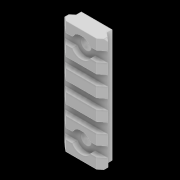
# Autodesk Inventor part: Picatinny6
Saved by Autodesk Inventor 2020.4 (Build 244396010, 396A)
## iProperties
Created: 2022-09-17
Part Number: Picatinny6
Material: Generic
Document SubType Name: Modeling
Designer: Val
Density: 1 g/cm^3
Appearance: Default
Author: Val
Autodesk Inventor part; units mm, degrees
ref_plane "YZ Plane" through (0, 0, 0) normal (1, 0, 0) x (0, 1, 0)
ref_plane "XZ Plane" through (0, 0, 0) normal (0, 1, 0) x (-1, 0, 0)
ref_plane "XY Plane" through (0, 0, 0) normal (0, 0, 1) x (1, 0, 0)
sketch "Base" plane through (0, 0, 0) normal (0, 0, 1) x (1, 0, 0)
  line L0 (-7.5, 55) -> (7.5, 55)
  line L1 (7.5, 55) -> (7.5, 0)
  line L2 (7.5, 0) -> (-7.5, 0)
  line L3 (-7.5, 0) -> (-7.5, 55)
  point P0 (0, 0)
  point P1 (0, 0)
  dimension "d0" = 55
  dimension "d1" = 15
  constraints: 8 end point, 2 parallel, 1 coincident, 1 horizontal, 1 midpoint, 1 perpendicular
  measures "d0" distance of L2.end L0.start
  measures "d1" distance of L0.start L0.end
extrude "BaseFeature" add sketch "Base" along normal blind 2.54
sketch "Profile" plane through (-7.5, 0, 0) normal (0, -1, 0) x (1, 0, 0)
  line L0 (0, 2.54) -> (15, 2.54) projected
  line L1 (0, 2.54) -> (15, 2.54)
  line L2 (15, 2.54) -> (15, 7.5692) construction
  line L3 (15, 7.5692) -> (0, 7.5692)
  line L4 (0, 7.5692) -> (0, 2.54) construction
  line L5 (-3.041, 5.0546) -> (18.041, 5.0546) construction
  line L6 (15, 7.5692) -> (18.041, 5.0546)
  line L7 (15, 2.54) -> (18.041, 5.0546)
  line L8 (0, 7.5692) -> (-3.041, 5.0546)
  line L9 (-3.041, 5.0546) -> (0, 2.54)
  point P0 (7.5, 0)
  point P1 (15, 5.0546)
  dimension "d4" = 5.0292
  dimension "d5" = 21.082
  constraints: 18 end point, 4 parallel, 2 horizontal, 1 midpoint, 1 perpendicular, 1 point on line
  measures "d4" distance of L0.end L2.end
  measures "d5" distance of L5.start L5.end
extrude "ProfileFeature" add sketch "Profile" against normal up to surface (55 mm away)
sketch "Rails" plane through (-7.5, 0, 7.5692) normal (0, 0, 1) x (1, 0, 0)
  line L0 (-3.041, 0) -> (-3.041, 55) projected
  line L1 (-3.041, 55) -> (18.041, 55)
  line L2 (18.041, 55) -> (18.041, 50)
  line L3 (18.041, 50) -> (-3.041, 50)
  line L4 (-3.041, 50) -> (-3.041, 55)
  line L5 (18.041, 0) -> (18.041, 55) projected
  line L6 (18.041, 40) -> (-3.041, 40)
  line L7 (-3.041, 45) -> (18.041, 45)
  line L8 (-3.041, 40) -> (-3.041, 45)
  line L9 (18.041, 45) -> (18.041, 40)
  line L10 (18.041, 30) -> (-3.041, 30)
  line L11 (-3.041, 35) -> (18.041, 35)
  line L12 (-3.041, 30) -> (-3.041, 35)
  line L13 (18.041, 35) -> (18.041, 30)
  line L14 (18.041, 20) -> (-3.041, 20)
  line L15 (-3.041, 25) -> (18.041, 25)
  line L16 (-3.041, 20) -> (-3.041, 25)
  line L17 (18.041, 25) -> (18.041, 20)
  line L18 (18.041, 10) -> (-3.041, 10)
  line L19 (-3.041, 15) -> (18.041, 15)
  line L20 (-3.041, 10) -> (-3.041, 15)
  line L21 (18.041, 15) -> (18.041, 10)
  line L22 (18.041, 0) -> (-3.041, 0)
  line L23 (-3.041, 5) -> (18.041, 5)
  line L24 (-3.041, 0) -> (-3.041, 5)
  line L25 (18.041, 5) -> (18.041, 0)
  point P0 (7.5, 0)
  point P1 (18.041, 0)
  point P2 (-3.041, 0)
  point P3 (18.041, 5)
  point P4 (18.041, 10)
  point P5 (-3.041, 10)
  point P6 (18.041, 15)
  point P7 (18.041, 20)
  point P8 (-3.041, 20)
  point P9 (18.041, 25)
  point P10 (18.041, 30)
  point P11 (-3.041, 30)
  point P12 (18.041, 35)
  point P13 (18.041, 40)
  point P14 (-3.041, 40)
  point P15 (18.041, 45)
  point P16 (18.041, 50)
  point P17 (-3.041, 50)
  point P18 (18.041, 55)
  dimension "d8" = 5
  dimension "d11" = 10
  constraints: 48 end point, 2 parallel, 1 collinear, 1 horizontal, 1 perpendicular, 1 vertical, 40 other
  measures "d8" distance between parallel lines of L1 L3
  measures "d11" distance of L2.end L6.start
extrude "RailsFeature" cut sketch "Rails" against normal up to surface (2.5146 mm away) contours L0 L18 L5 L23 | L0 L14 L5 L19 | L0 L10 L5 L15 | L0 L6 L5 L11 | L0 L3 L5 L7
sketch "Corners" plane through (0, 0, 0) normal (0, 0, -1) x (-1, 0, 0)
  line L0 (-10.541, 55) -> (-7.5, 55) projected
  line L1 (-10.541, 55) -> (-9.4234, 55)
  line L2 (-9.4234, 55) -> (-9.4234, 53.8824)
  line L3 (-9.4234, 53.8824) -> (-10.541, 53.8824)
  line L4 (-10.541, 53.8824) -> (-10.541, 55)
  line L5 (0, -19) -> (0, 114) construction
  line L6 (10.541, 55) -> (9.4234, 55)
  line L7 (9.4234, 55) -> (9.4234, 53.8824)
  line L8 (9.4234, 53.8824) -> (10.541, 53.8824)
  line L9 (10.541, 53.8824) -> (10.541, 55)
  line L10 (-7.5, 55) -> (7.5, 55) construction
  line L11 (0, 55) -> (0, 0) construction
  line L12 (0, 27.5) -> (10.541, 27.5) construction
  line L13 (-10.541, 0) -> (-9.4234, 0)
  line L14 (-9.4234, 0) -> (-9.4234, 1.1176)
  line L15 (-9.4234, 1.1176) -> (-10.541, 1.1176)
  line L16 (-10.541, 1.1176) -> (-10.541, 0)
  line L17 (10.541, 0) -> (9.4234, 0)
  line L18 (10.541, 1.1176) -> (10.541, 0)
  line L19 (9.4234, 0) -> (9.4234, 1.1176)
  line L20 (9.4234, 1.1176) -> (10.541, 1.1176)
  line L21 (-10.541, 53.8824) -> (-9.4234, 55)
  line L22 (9.4234, 55) -> (10.541, 53.8824)
  line L23 (9.4234, 0) -> (10.541, 1.1176)
  line L24 (-10.541, 1.1176) -> (-9.4234, 0)
  dimension "d36" = 1.1176
  constraints: 44 end point, 12 symmetric about line, 6 perpendicular, 2 horizontal, 2 midpoint, 2 parallel
  measures "d36" distance of L2.end L3.end
extrude "CornersFeature" cut sketch "Corners" against normal through all contours L0 L21 L4 | L9 L22 L6 | L16 L24 L13 | L17 L23 L18
sketch "MountHoles" plane through (-10.541, 40, 5.0546) normal (0, 0, 1) x (1, 0, 0)
  line L0 (0, 0) -> (21.082, 0) construction
  line L1 (0, -5) -> (0, 0) construction
  line L2 (21.082, -5) -> (0, -5) construction
  line L3 (21.082, -5) -> (21.082, 0) construction
  line L4 (21.082, 5) -> (21.082, 10) construction
  line L5 (0, -10) -> (21.082, -10) projected
  line L6 (0, -15) -> (0, -10) projected
  line L7 (21.082, -15) -> (0, -15) projected
  line L8 (21.082, -15) -> (21.082, -10) projected
  line L9 (0, -20) -> (21.082, -20) projected
  line L10 (0, -25) -> (0, -20) projected
  line L11 (21.082, -25) -> (0, -25) projected
  line L12 (21.082, -25) -> (21.082, -20) projected
  line L13 (0, 0) -> (21.082, 0) projected
  line L14 (0, -5) -> (0, 0) projected
  line L15 (21.082, -5) -> (0, -5) projected
  line L16 (21.082, -5) -> (21.082, 0) projected
  line L17 (0, -30) -> (21.082, -30) projected
  line L18 (0, -35) -> (0, -30) projected
  line L19 (21.082, -35) -> (0, -35) projected
  line L20 (21.082, -35) -> (21.082, -30) projected
  line L21 (0, 10) -> (21.082, 10) projected
  line L22 (0, 5) -> (0, 10) projected
  line L23 (21.082, 5) -> (0, 5) projected
  circle A0 centre (10.541, 7.5) radius 2.5
  circle A1 centre (10.541, -32.5) radius 2.5
  line L24 (3.041, 10) -> (18.041, 10) projected
  line L25 (18.041, 5) -> (3.041, 5) projected
  line L26 (18.041, 15) -> (3.041, 15) projected
  line L27 (10.541, 15) -> (10.541, -40) construction
  line L28 (18.041, -40) -> (3.041, -40) projected
  line L29 (3.041, -30) -> (18.041, -30) projected
  line L30 (18.041, -35) -> (3.041, -35) projected
  constraints: 5 tangent, 2 centre point, 2 end point, 2 midpoint, 2 point on line
hole "MountHolesFeature" at (0, 47.5, 5.0546) at (0, 7.5, 5.0546) direction (0, 0, -1) diameter 5 depth 25.4 tip angle 118
sketch "Countersinks" plane through (-10.541, 15, 5.0546) normal (0, 0, 1) x (1, 0, 0)
  arc A0 (10.541, 30) -> (10.541, 35) centre (10.541, 32.5) ccw construction
  arc A1 (10.541, -10) -> (10.541, -5) centre (10.541, -7.5) ccw construction
  circle A2 centre (10.541, 32.5) radius 5
  circle A3 centre (10.541, -7.5) radius 5
  dimension "d39" = 10
  constraints: 2 centre point, 2 coincident, 1 equal radius
  measures "d39" diameter of A2
extrude "CountersinksFeature" cut sketch "Countersinks" along normal through all
sketch "Spacers" plane through (0, 0, 0) normal (0, 0, -1) x (-1, 0, 0)
  line L0 (10.541, 35) -> (10.541, 40) projected
  circle A0 centre (0, 47.5) radius 2.5 projected
  circle A1 centre (0, 7.5) radius 2.5 projected
  circle A2 centre (0, 47.5) radius 2.5 projected
  circle A3 centre (0, 47.5) radius 4.5
  circle A4 centre (0, 7.5) radius 4.5
  point P0 (0, 117.5)
  dimension "d41" = 2
  constraints: 2 centre point, 2 coincident, 1 equal radius
  measures "d41" radial gap between concentric circles of A3 A0
extrude "SpacersFeature" add sketch "Spacers" along normal blind 1
body "Solid1"
